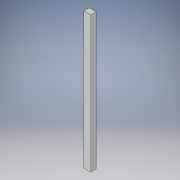
# Autodesk Inventor part: slider
Saved by Autodesk Inventor 2019 (Build 230136000, 136)
## iProperties
Created: 2019-10-13
Part Number: slider
Material: Generic
Document SubType Name: Modeling
Designer: hp
Density: 1 g/cm^3
Appearance: Default
Author: hp
Autodesk Inventor part; units mm, degrees
ref_plane "YZ Plane" through (0, 0, 0) normal (1, 0, 0) x (0, 1, 0)
ref_plane "XZ Plane" through (0, 0, 0) normal (0, 1, 0) x (-1, 0, 0)
ref_plane "XY Plane" through (0, 0, 0) normal (0, 0, 1) x (1, 0, 0)
sketch "Sketch1" plane through (0, 0, 0) normal (1, 0, 0) x (0, 1, 0)
  line L0 (8.2852, 7.4086) -> (8.2852, 7.0127)
  line L1 (8.2852, 7.0127) -> (-1.838, 7.0127)
  line L2 (-1.838, 7.0127) -> (-1.838, 7.4086)
  line L3 (-1.838, 7.4086) -> (8.2852, 7.4086)
  point P0 (0, 0)
  constraints: 8 end point, 3 perpendicular, 1 vertical
extrude "Extrusion1" add sketch "Sketch1" along normal blind 0.5
body "Solid1"
